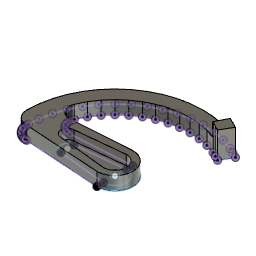
Smart_Useless_Box_lid_arm_v2 (Autodesk Fusion 360 design; units mm, degrees)
Autodesk Fusion 360 part; units mm, degrees
other "Base Mesh Feature1"
imported_body "Base Feature1" makes body 1
sketch "sketch 210" plane through (0, 0, 0) normal (0, 0, 1) x (1, 0, 0)
  line L0 (-7.9205, 16.4366) -> (-5.5919, 19.0919)
  line L1 (-9.8827, 13.5) -> (-7.9205, 16.4366)
  line L2 (-7.9942, 7.7233) -> (-7.9175, 8.2729)
  line L3 (-2.9366, 21.4205) -> (0, 23.3827)
  line L4 (6.5119, 26.08) -> (9.9758, 26.769)
  line L5 (-7.9942, 7.7233) -> (-7.9773, 7.1686)
  line L6 (-0.5015, 18.2471) -> (2, 19.9186)
  line L7 (-7.9773, 7.1686) -> (-7.8671, 6.6247)
  line L8 (-11.4447, 10.3325) -> (-9.8827, 13.5)
  line L9 (-11.5, -3.4641) -> (-11.0307, -3.6955)
  line L10 (-7.3823, 5.6308) -> (-7.0215, 5.2091)
  line L11 (-12.3284, -2.8284) -> (-11.935, -3.1734)
  line L12 (-9.5, -4) -> (13.5, -5.5)
  line L13 (-7.7492, 8.8017) -> (-6.4186, 11.5)
  line L14 (13.5, 23) -> (16.5021, 22.8032)
  line L15 (-7.6669, 6.1072) -> (-7.3823, 5.6308)
  line L16 (-7.0215, 5.2091) -> (-6.5948, 4.8543)
  line L17 (-6.5948, 4.8543) -> (-6.1145, 4.5765)
  line L18 (-13.5, 0) -> (-13.4658, 0.5221)
  line L19 (0, 23.3827) -> (3.1675, 24.9447)
  line L20 (3.1675, 24.9447) -> (6.5119, 26.08)
  line L21 (4.6983, 21.2492) -> (7.5472, 22.2163)
  line L22 (19.4528, 22.2163) -> (22.3017, 21.2492)
  line L23 (-5.0488, 4.281) -> (-4.4939, 4.2718)
  line L24 (-4.4939, 4.2718) -> (13.5, 5.5)
  line L25 (-6.4186, 11.5) -> (-4.7471, 14.0015)
  line L26 (13.5, 27) -> (17.0242, 26.769)
  line L27 (-12.58, 6.9881) -> (-11.4447, 10.3325)
  line L28 (-13.5, 0) -> (-13.4658, -0.5221)
  line L29 (-11.0307, -3.6955) -> (-10.5353, -3.8637)
  line L30 (-13.269, 3.5242) -> (-12.58, 6.9881)
  line L31 (-6.1145, 4.5765) -> (-5.5941, 4.3835)
  line L32 (25, 19.9186) -> (27, 23.3827)
  line L33 (-10.0221, -3.9658) -> (-9.5, -4)
  line L34 (7.5472, 22.2163) -> (10.4979, 22.8032)
  line L35 (-2.7635, 16.2635) -> (-0.5015, 18.2471)
  line L36 (23.8325, 24.9447) -> (25.4162, 24.1637)
  line L37 (25.4162, 24.1637) -> (27, 23.3827)
  line L38 (-11.935, -3.1734) -> (-11.5, -3.4641)
  line L39 (-13.4658, 0.5221) -> (-13.269, 3.5242)
  line L40 (23.6509, 20.5839) -> (25, 19.9186)
  line L41 (22.3017, 21.2492) -> (23.6509, 20.5839)
  line L42 (-5.5941, 4.3835) -> (-5.0488, 4.281)
  line L43 (-12.9641, -2) -> (-12.6734, -2.435)
  line L44 (-5.5919, 19.0919) -> (-2.9366, 21.4205)
  line L45 (-7.9175, 8.2729) -> (-7.7492, 8.8017)
  line L46 (17.0242, 26.769) -> (20.4881, 26.08)
  line L47 (-7.8671, 6.6247) -> (-7.6669, 6.1072)
  line L48 (20.4881, 26.08) -> (23.8325, 24.9447)
  line L49 (2, 19.9186) -> (4.6983, 21.2492)
  line L50 (-4.7471, 14.0015) -> (-2.7635, 16.2635)
  line L51 (16.5021, 22.8032) -> (19.4528, 22.2163)
  line L52 (-10.5353, -3.8637) -> (-10.0221, -3.9658)
  line L53 (10.4979, 22.8032) -> (13.5, 23)
  line L54 (9.9758, 26.769) -> (13.5, 27)
  line L55 (-13.4658, -0.5221) -> (-13.3637, -1.0353)
  line L56 (-13.3637, -1.0353) -> (-13.1955, -1.5307)
  line L57 (-13.1955, -1.5307) -> (-12.9641, -2)
  line L58 (-12.6734, -2.435) -> (-12.3284, -2.8284)
  line L59 (-1, 2) -> (13.5, 3.5)
  line L60 (-1, -2) -> (13.5, -3.5)
  circle A0 centre (13.5072, 0.0041) radius 1
  arc A1 (13.5, -3.5) -> (13.5, 3.5) centre (13.5, 0) ccw
  arc A2 (13.5, -5.5) -> (13.5, 5.5) centre (13.5, 0) ccw
  arc A3 (-1, 2) -> (-1, -2) centre (-1, 0) ccw
  constraint coincident L59.end A1.end
  constraint coincident L60.end A1.start
  constraint coincident L24.end A2.end
  constraint coincident L12.end A2.start
  constraint coincident L59.start A3.start
  constraint coincident L60.start A3.end
extrude "Extrude1" add sketch "sketch 210" along normal blind 1 separate body contours L59 L60 A1 A3 makes body 2
extrude "Extrude2" add sketch "sketch 210" along normal blind 4 contours L0 L1 L2 L3 L4 L5 L6 L7 L8 L9 L10 L11 L12 L13 L14 L15 L16 L17 L18 L19 L20 L21 L22 L23 L24 L25 L26 L27 L28 L29 L30 L31 L32 L33 L34 L35 L36 L37 L38 L39 L40 L41 L42 L43 L44 L45 L46 L47 L48 L49 L50 L51 L52 L53 L54 L55 L56 L57 L58 A2 bodies 2
chamfer "Chamfer1" distance 1 angle 45 1 edges at (12.5748, 0.3657, 0) on bodies 2
sketch "Sketch1" plane through (0, 0, 4) normal (0, 0, 1) x (-1, 0, 0)
  arc A0 (1, -2) -> (1, 2) centre (1, 0) ccw
  line L0 (1, -2) -> (-13.5, -3.5)
  arc A1 (-13.5, 3.5) -> (-13.5, -3.5) centre (-13.5, 0) ccw
  line L1 (-13.5, 3.5) -> (1, 2)
  line L2 (13.5, 0) -> (13.4658, 0.5221)
  line L3 (13.4658, 0.5221) -> (13.3637, 1.0353)
  line L4 (13.3637, 1.0353) -> (13.1955, 1.5307)
  line L5 (13.1955, 1.5307) -> (12.9641, 2)
  line L6 (12.9641, 2) -> (12.6734, 2.435)
  line L7 (12.6734, 2.435) -> (12.3284, 2.8284)
  line L8 (12.3284, 2.8284) -> (11.935, 3.1734)
  line L9 (11.935, 3.1734) -> (11.5, 3.4641)
  line L10 (11.5, 3.4641) -> (11.0307, 3.6955)
  line L11 (11.0307, 3.6955) -> (10.5353, 3.8637)
  line L12 (10.5353, 3.8637) -> (10.0221, 3.9658)
  line L13 (10.0221, 3.9658) -> (9.5, 4)
  line L14 (9.5, 4) -> (-13.5, 5.5)
  arc A2 (-13.5, 5.5) -> (-13.5, -5.5) centre (-13.5, 0) ccw
  line L15 (-13.5, -5.5) -> (4.4939, -4.2718)
  line L16 (4.4939, -4.2718) -> (5.0488, -4.281)
  line L17 (5.0488, -4.281) -> (5.5941, -4.3835)
  line L18 (5.5941, -4.3835) -> (6.1145, -4.5765)
  line L19 (6.1145, -4.5765) -> (6.5948, -4.8543)
  line L20 (6.5948, -4.8543) -> (7.0215, -5.2091)
  line L21 (7.0215, -5.2091) -> (7.3823, -5.6308)
  line L22 (7.3823, -5.6308) -> (7.6669, -6.1072)
  line L23 (7.6669, -6.1072) -> (7.8671, -6.6247)
  line L24 (7.8671, -6.6247) -> (7.9773, -7.1686)
  line L25 (7.9773, -7.1686) -> (7.9942, -7.7233)
  line L26 (7.9942, -7.7233) -> (7.9175, -8.2729)
  line L27 (7.9175, -8.2729) -> (7.7492, -8.8017)
  line L28 (7.7492, -8.8017) -> (6.4186, -11.5)
  line L29 (6.4186, -11.5) -> (4.7471, -14.0015)
  line L30 (4.7471, -14.0015) -> (2.7635, -16.2635)
  line L31 (2.7635, -16.2635) -> (0.5015, -18.2471)
  line L32 (0.5015, -18.2471) -> (-2, -19.9186)
  line L33 (-2, -19.9186) -> (-4.6983, -21.2492)
  line L34 (-4.6983, -21.2492) -> (-7.5472, -22.2163)
  line L35 (-7.5472, -22.2163) -> (-10.4979, -22.8032)
  line L36 (-10.4979, -22.8032) -> (-13.5, -23)
  line L37 (-13.5, -23) -> (-16.5021, -22.8032)
  line L38 (-16.5021, -22.8032) -> (-19.4528, -22.2163)
  line L39 (-19.4528, -22.2163) -> (-22.3017, -21.2492)
  line L40 (-22.3017, -21.2492) -> (-23.6509, -20.5839)
  line L41 (-23.6509, -20.5839) -> (-25, -19.9186)
  line L42 (-25, -19.9186) -> (-27, -23.3827)
  line L43 (-27, -23.3827) -> (-23.8325, -24.9447)
  line L44 (-23.8325, -24.9447) -> (-20.4881, -26.08)
  line L45 (-20.4881, -26.08) -> (-17.0242, -26.769)
  line L46 (-17.0242, -26.769) -> (-13.5, -27)
  line L47 (-13.5, -27) -> (-9.9758, -26.769)
  line L48 (-9.9758, -26.769) -> (-6.5119, -26.08)
  line L49 (-6.5119, -26.08) -> (-3.1675, -24.9447)
  line L50 (-3.1675, -24.9447) -> (0, -23.3827)
  line L51 (0, -23.3827) -> (2.9366, -21.4205)
  line L52 (2.9366, -21.4205) -> (5.5919, -19.0919)
  line L53 (5.5919, -19.0919) -> (7.9205, -16.4366)
  line L54 (7.9205, -16.4366) -> (9.8827, -13.5)
  line L55 (9.8827, -13.5) -> (11.4447, -10.3325)
  line L56 (11.4447, -10.3325) -> (12.58, -6.9881)
  line L57 (12.58, -6.9881) -> (13.269, -3.5242)
  line L58 (13.269, -3.5242) -> (13.4658, -0.5221)
  line L59 (13.4658, -0.5221) -> (13.5, 0)
  line L60 (-23.8325, -24.9447) -> (-22.0519, -21.334)
  line L61 (-25, -19.9186) -> (-27, -23.3827)
  line L62 (-23.8325, -24.9447) -> (-27, -23.3827)
  constraint coincident L43.end L44.start
  constraint coincident L39 L60.end
  constraint perpendicular L40 L60
  constraint coincident L41.end L42.start
  constraint coincident L42.end L43.start
extrude "Extrude3" add sketch "Sketch1" along normal blind 4 contours L39 L40 L41 L42 L43 L60 L61 L62 bodies 2
hidden bodies 1
